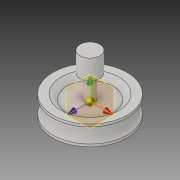
# Autodesk Inventor part: Top Spoolish
Saved by Autodesk Inventor 2018 (Build 220112000, 112)
## iProperties
Created: 2017-12-12
Part Number: Top Spoolish
Material: Generic
Document SubType Name: Modeling
Designer: Rus
Density: 1 g/cm^3
Appearance: Default
Mass: 18.9348 g
Surface Area: 68.2841 cm^2
Volume: 18.9348 cm^3
Author: Rus
Autodesk Inventor part; units mm, degrees
ref_plane "YZ Plane" through (0, 0, 0) normal (1, 0, 0) x (0, 1, 0)
ref_plane "XZ Plane" through (0, 0, 0) normal (0, 1, 0) x (-1, 0, 0)
ref_plane "XY Plane" through (0, 0, 0) normal (0, 0, 1) x (1, 0, 0)
sketch "Sketch1" plane through (0, 0, 0) normal (0, 0, 1) x (1, 0, 0)
  line L0 (0, 0) -> (0, 21.1667)
  line L1 (0, 0) -> (0, -10.5833)
  line L2 (0, 21.1667) -> (0, 33.8667)
  line L3 (6.35, 21.1667) -> (6.35, 33.8667)
  line L4 (6.35, 33.8667) -> (0, 33.8667)
  line L5 (3.175, 12.7991) -> (0, 12.7991) construction
  line L6 (6.35, 21.1667) -> (3.175, 21.1667)
  line L7 (3.175, 21.1667) -> (0, 21.1667) construction
  line L8 (0, 0) -> (3.175, 0) construction
  line L9 (3.175, 0) -> (17.91, 0) construction
  line L10 (23.8125, 7.9375) -> (23.8125, 9.525)
  line L11 (14.8167, 6.35) -> (3.175, 6.35)
  line L12 (18.6267, 9.525) -> (23.8125, 9.525)
  line L13 (0, -10.5833) -> (3.175, -8.4667)
  line L14 (3.175, -8.4667) -> (3.175, 0)
  line L15 (14.8167, 6.35) -> (18.6267, 9.525)
  line L16 (3.175, 21.1667) -> (3.175, 6.35)
  line L17 (1.0583, 6.35) -> (3.175, 6.35) construction
  line L18 (1.0583, 6.35) -> (1.0583, 3.175) construction
  line L19 (1.0583, 3.175) -> (5.214, 3.175) construction
  line L20 (23.8125, -1.5875) -> (23.8125, -3.175)
  line L21 (14.8167, 0) -> (3.175, 0)
  line L22 (18.6267, -3.175) -> (23.8125, -3.175)
  line L23 (14.8167, 0) -> (18.6267, -3.175)
  line L24 (3.175, 0) -> (3.175, 0)
  arc A0 (23.8125, 7.9375) -> (23.8125, -1.5875) centre (30.8127, 3.175) ccw
  line L25 (23.8125, -3.175) -> (23.495, -3.175)
  dimension "d5" = 44.45
  dimension "d6" = 12.7
  dimension "d7" = 6.35
  dimension "d12" = 2.1167
  dimension "d13" = 3.175
  dimension "d15" = 8.4667
  dimension "d18" = 1.5875
  dimension "d20" = 3.175
  dimension "d21" = 3.81
  dimension "d26" = 23.8125
  dimension "d30" = 11.6417
  dimension "d31" = 3.175
  dimension "d32" = 2.1167
  dimension "d33" = 8.4667
  dimension "d34" = 3.175
  dimension "d36" = 0.3175
  constraints: 53 end point, 7 vertical, 6 horizontal, 5 symmetric about line, 4 point on line, 3 perpendicular, 2 point on circle, 1 centre point
  measures "d5" distance of L2.end L1.end
  measures "d6" distance of L3.start L3.end
  measures "d7" distance between parallel lines of L2 L3
  measures "d12" vertical distance of L13.end L1.end
  measures "d13" horizontal distance of L1.end L13.end
  measures "d15" distance from line of L9 L13.end
  measures "d18" distance of L10.end L10.start
  measures "d20" distance between parallel lines of L11 L12
  measures "d21" horizontal distance of L12.start L11.start
  measures "d26" horizontal distance of L10.start L1.end
  measures "d30" distance of L11.start L11.end
  measures "d31" distance of L17.start L18.end
  measures "d32" distance of L17.start L11.end
  measures "d33" radius of A0
  measures "d34" distance of L6.end L0.end
  measures "d36" distance of L22.end L25.end
revolve "Revolution1" add sketch "Sketch1" angle 360 about axis through (0, 21.1667, 0) along (0, -1, 0)
move faces "Move1" translate (0, -1.27, 0) faces at (10.7618, 0, -1.4352)
body "Solid1"
